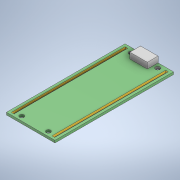
# Autodesk Inventor part: RaspPi-Pico
Saved by Autodesk Inventor 2022 (Build 260153000, 153)
## iProperties
Created: 2022-10-11
Part Number: RaspPi-Pico
Material: Generic
Document SubType Name: Modeling
Designer: richb366163
Density: 1 g/cm^3
Appearance: Default
Author: richb366163
Autodesk Inventor part; units mm, degrees
ref_plane "YZ Plane" through (0, 0, 0) normal (1, 0, 0) x (0, 1, 0)
ref_plane "XZ Plane" through (0, 0, 0) normal (0, 1, 0) x (-1, 0, 0)
ref_plane "XY Plane" through (0, 0, 0) normal (0, 0, 1) x (1, 0, 0)
sketch "Sketch1" plane through (0, 0, 0) normal (0, 1, 0) x (-1, 0, 0)
  line L0 (0, 0) -> (21.0058, 0)
  line L1 (21.0058, 0) -> (21.0058, -51.308)
  line L2 (21.0058, -51.308) -> (0, -51.308)
  line L3 (0, -51.308) -> (0, 0)
  line L4 (21.0058, -51.308) -> (19.8628, -51.308)
  line L5 (19.8628, -51.308) -> (19.8628, -50.292)
  line L6 (19.8628, -50.292) -> (21.0058, -50.292)
  line L7 (21.0058, -50.292) -> (21.0058, -51.308)
  line L8 (21.0058, -25.654) -> (0, -25.654)
  line L9 (10.5029, -51.308) -> (10.5029, 0)
  line L10 (19.8628, 0) -> (19.8628, -1.016)
  line L11 (19.8628, -1.016) -> (21.0058, -1.016)
  line L12 (1.143, -51.308) -> (1.143, -50.292)
  line L13 (1.143, -50.292) -> (0, -50.292)
  line L14 (1.143, -1.016) -> (0, -1.016)
  line L15 (1.143, 0) -> (1.143, -1.016)
  line L16 (19.8628, -1.016) -> (19.8628, -50.292)
  line L17 (19.8628, -50.292) -> (18.7198, -50.292)
  line L18 (18.7198, -50.292) -> (18.7198, -1.016)
  line L19 (18.7198, -1.016) -> (19.8628, -1.016)
  line L20 (1.143, -1.016) -> (1.143, -50.292)
  line L21 (1.143, -50.292) -> (2.286, -50.292)
  line L22 (2.286, -50.292) -> (2.286, -1.016)
  line L23 (2.286, -1.016) -> (1.143, -1.016)
  line L24 (21.0058, 0) -> (17.1958, 0)
  line L25 (17.1958, 0) -> (17.1958, -0.9398)
  line L26 (17.1958, -0.9398) -> (21.0058, -0.9398)
  line L27 (21.0058, -0.9398) -> (21.0058, 0)
  line L28 (17.1958, -0.9398) -> (15.2908, -0.9398)
  line L29 (15.2908, -0.9398) -> (15.2908, -2.8448)
  line L30 (15.2908, -2.8448) -> (17.1958, -2.8448)
  line L31 (17.1958, -2.8448) -> (17.1958, -0.9398)
  circle A0 centre (16.2433, -1.8923) radius 0.9525
  circle A1 centre (4.7625, -1.8923) radius 0.9525
  line L32 (21.0058, -51.308) -> (0, -51.308)
  line L33 (0, -51.308) -> (0, -50.165)
  line L34 (0, -50.165) -> (21.0058, -50.165)
  line L35 (21.0058, -50.165) -> (21.0058, -51.308)
  line L36 (21.0058, -50.165) -> (17.1958, -50.165)
  line L37 (17.1958, -50.165) -> (15.2908, -50.165)
  line L38 (15.2908, -50.165) -> (15.2908, -48.26)
  line L39 (15.2908, -48.26) -> (17.1958, -48.26)
  line L40 (17.1958, -48.26) -> (17.1958, -50.165)
  circle A2 centre (16.2433, -49.2125) radius 0.9525
  circle A3 centre (4.7625, -49.2125) radius 0.9525
  point P0 (19.8628, -50.165)
  point P1 (18.7198, -50.165)
  point P2 (2.286, -50.165)
  point P3 (1.143, -50.165)
  dimension "d0" = 21.0058
  dimension "d1" = 51.308
  dimension "d2" = 1.143
  dimension "d3" = 1.016
  dimension "d4" = 1.143
  dimension "d7" = 3.81
  dimension "d8" = 0.9398
  dimension "d9" = 1.905
  dimension "d10" = 1.905
  dimension "d11" = 1.143
  dimension "d12" = 3.81
  dimension "d13" = 1.905
  dimension "d14" = 1.905
  constraints: 82 end point, 15 parallel, 13 symmetric about line, 7 perpendicular, 6 horizontal, 4 centre point, 4 midpoint, 2 point on line, 2 other
  measures "d0" distance of L1.end L2.end
  measures "d1" distance of L0.end L1.end
  measures "d2" distance of L5.end L6.end
  measures "d3" distance of L4.end L5.end
  measures "d4" distance of L5.end L17.end
  measures "d7" distance of L26.end L25.end
  measures "d8" distance of L25.end L24.end
  measures "d9" distance of L30.end L29.end
  measures "d10" distance of L29.end L28.end
  measures "d11" distance of L32.end L33.end
  measures "d12" distance of L34.end L36.end
  measures "d13" distance of L38.end L39.end
  measures "d14" distance of L37.end L38.end
extrude "Extrusion1" add sketch "Sketch1" along normal blind 1.016 contours L0 L15 L14 L3 | L0 L9 L8 L22 L23 L15 | L14 L20 L8 L3 | L31 A0 L28 | L0 L25 L26 L10 L19 L18 L8 L9 | L8 L20 L34 L3 | L0 L10 L26 L25 | L9 L34 L22 L8 | L8 L18 L34 L40 L39 L38 L9 | L34 L20 L13 L3 | L0 L1 L26 L10 | L34 L18 L17 L5 L2 L9 | L9 L2 L12 L21 L22 L34 | L34 L22 L21 L20 | L13 L12 L2 L3 | L26 L1 L11 L10 | A0 L29 L28 | L31 L30 A0 | L16 L11 L1 L8 | L8 L1 L34 L16 | L34 L16 L17 L18 | L38 A2 L34 | A0 L30 L29 | L34 L1 L6 L16 | L34 A2 L40 | L5 L6 L1 L2 | L38 L39 A2 | A2 L39 L40
sketch "Sketch2" plane through (0, 1.016, 0) normal (0, 1, 0) x (1, 0, 0)
  line L0 (0, 51.308) -> (-21.0058, 51.308) projected
  line L1 (-10.5029, 51.308) -> (-14.2875, 51.308)
  line L2 (-14.2875, 51.308) -> (-14.2875, 49.2125)
  line L3 (-14.2875, 49.2125) -> (-10.5029, 49.2125)
  line L4 (-10.5029, 49.2125) -> (-10.5029, 51.308)
  line L5 (-21.0058, 51.308) -> (0, 51.308)
  line L6 (-6.7183, 51.308) -> (-6.7183, 49.2125)
  line L7 (-6.7183, 49.2125) -> (-10.5029, 49.2125)
  point P0 (0, 0)
  constraints: 14 end point, 4 symmetric about line, 2 parallel, 1 horizontal, 1 midpoint, 1 perpendicular
extrude "Extrusion2" add sketch "Sketch2" along normal blind 2.54
sketch "Sketch3" plane through (-14.2875, 1.016, -49.2125) normal (0, 0, 1) x (1, 0, 0)
  line L0 (0, 2.54) -> (7.5692, 2.54) projected
  line L1 (7.5692, 0) -> (0, 0) projected
  line L2 (0, 2.54) -> (7.5692, 2.54)
  line L3 (7.5692, 2.54) -> (7.5692, 0)
  line L4 (7.5692, 0) -> (0, 0)
  line L5 (0, 0) -> (0, 2.54)
  point P0 (14.2875, -1.016)
  constraints: 8 end point, 2 parallel, 1 horizontal, 1 perpendicular
extrude "Extrusion3" add sketch "Sketch3" along normal blind 2.54
body "Solid1"
